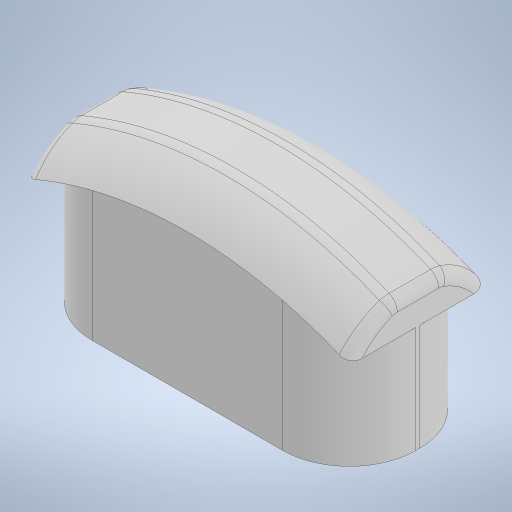
# Autodesk Inventor part: гриб
Saved by Autodesk Inventor 2023.1 (Build 271208000, 208)
## iProperties
Created: 2024-12-27
Part Number: гриб
Material: Типовые
Document SubType Name: Modeling
Designer: DELL
Density: 1 g/cm^3
Appearance: По умолчанию
Author: DELL
Autodesk Inventor part; units mm, degrees
ref_plane "YZ Plane" through (0, 0, 0) normal (1, 0, 0) x (0, 1, 0)
ref_plane "XZ Plane" through (0, 0, 0) normal (0, 1, 0) x (-1, 0, 0)
ref_plane "XY Plane" through (0, 0, 0) normal (0, 0, 1) x (1, 0, 0)
sketch "Эскиз1" plane through (0, 0, 0) normal (0, 1, 0) x (-1, 0, 0)
  line L0 (7.15, 2.15) -> (-7.15, 2.15)
  line L1 (-9.15, 0.15) -> (-9.15, -0.15)
  line L2 (-7.15, -2.15) -> (7.15, -2.15)
  line L3 (9.15, -0.15) -> (9.15, 0.15)
  line L4 (9.15, 2.15) -> (-9.15, -2.15) construction
  line L5 (-9.15, 2.15) -> (9.15, -2.15) construction
  arc A0 (-7.15, 2.15) -> (-9.15, 0.15) centre (-7.15, 0.15) ccw
  arc A1 (-9.15, -0.15) -> (-7.15, -2.15) centre (-7.15, -0.15) ccw
  arc A2 (9.15, 0.15) -> (7.15, 2.15) centre (7.15, 0.15) ccw
  arc A3 (7.15, -2.15) -> (9.15, -0.15) centre (7.15, -0.15) ccw
  line L6 (7.15, -5.15) -> (-7.15, -5.15)
  arc A4 (-12.15, -0.15) -> (-7.15, -5.15) centre (-7.15, -0.15) ccw
  line L7 (-12.15, -0.15) -> (-12.15, 0.15)
  arc A5 (-7.15, 5.15) -> (-12.15, 0.15) centre (-7.15, 0.15) ccw
  line L8 (-7.15, 5.15) -> (7.15, 5.15)
  arc A6 (12.15, 0.15) -> (7.15, 5.15) centre (7.15, 0.15) ccw
  line L9 (12.15, 0.15) -> (12.15, -0.15)
  arc A7 (7.15, -5.15) -> (12.15, -0.15) centre (7.15, -0.15) ccw
  point P0 (0, 0)
  dimension "d0" = 18.3
  dimension "d1" = 4.3
  dimension "d2" = 2
  dimension "d3" = 3
  constraints: 20 end point, 16 point on circle, 8 centre point, 8 point on line, 8 tangent, 4 parallel, 3 equal radius, 2 midpoint, 2 perpendicular, 1 horizontal, 7 other
  measures "d0" distance of L4.end L5.end
  measures "d1" distance of L5.start L4.end
  measures "d2" radius of A0
  measures "d3" distance between parallel lines of L2 L6
extrude "Выдавливание1" add sketch "Эскиз1" along normal blind 8
sketch "Эскиз2" plane through (12.15, 0, 0.15) normal (1, 0, 0) x (0, 0, -1)
  line L0 (0, 0) -> (0, 8) construction
  line L1 (0, 8) -> (0.3, 8) construction
  line L2 (0.3, 0) -> (0.3, 8) construction
  line L3 (0.3, 0) -> (0, 0) construction
  line L4 (-5, 0) -> (-5, 8) construction
  line L5 (5.3, 8) -> (0.3, 8) projected
  line L6 (-5, 8) -> (5.3, 8)
  line L7 (-1.4023, 10.3381) -> (1.7023, 10.3381)
  arc A0 (5.3, 8) -> (2.4133, 10.2075) centre (0.15, 4.2565) ccw
  arc A1 (-2.1133, 10.2075) -> (-5, 8) centre (0.15, 4.2565) ccw
  arc A2 (-1.4023, 10.3381) -> (-2.1133, 10.2075) centre (-1.4023, 8.3381) ccw
  arc A3 (2.4133, 10.2075) -> (1.7023, 10.3381) centre (1.7023, 8.3381) ccw
  point P0 (-1.7343, 10.3381)
  point P1 (2.0343, 10.3381)
  dimension "d6" = 2
  constraints: 14 end point, 10 point on circle, 4 centre point, 4 tangent, 2 horizontal, 2 point on line, 1 equal radius
  measures "d6" radius of A2
ref_plane "РабПлоскость1" through (-7.15, 0, 0) normal (0, 0, 1) x (1, 0, 0)
sketch "Эскиз3" plane through (-7.15, 0, 0) normal (0, 0, 1) x (1, 0, 0)
  line L0 (19.3, 8) -> (19.3, 10.2075) construction
  line L1 (0, 0) -> (-5, 0) projected
  line L2 (-5, 0) -> (-5, 15.3004) construction
  arc A0 (19.3, 9.1037) -> (-5, 9.1037) centre (7.15, -17.7297) ccw
  point P0 (7.15, 0)
  constraints: 2 end point, 2 point on circle, 1 centre point, 1 midpoint, 1 point on line, 1 vertical
sweep "Сдвиг1" add profiles "Эскиз2" path "Эскиз3" keep normal constant yes path curves A0
sketch "Эскиз4" plane through (0, 8, 0) normal (0, 1, 0) x (1, 0, 0)
  line L0 (-7.15, -5.15) -> (7.15, -5.15)
  arc A0 (-12.15, -0.15) -> (-7.15, -5.15) centre (-7.15, -0.15) ccw
  line L1 (-12.15, 0.15) -> (-12.15, -0.15)
  arc A1 (-7.15, 5.15) -> (-12.15, 0.15) centre (-7.15, 0.15) ccw
  line L2 (7.15, 5.15) -> (-7.15, 5.15)
  arc A2 (12.15, 0.15) -> (7.15, 5.15) centre (7.15, 0.15) ccw
  line L3 (12.15, -0.15) -> (12.15, 0.15)
  arc A3 (7.15, -5.15) -> (12.15, -0.15) centre (7.15, -0.15) ccw
  arc A4 (-9.15, -0.15) -> (-7.15, -2.15) centre (-7.15, -0.15) ccw
  line L4 (7.15, -2.15) -> (-7.15, -2.15)
  arc A5 (7.15, -2.15) -> (9.15, -0.15) centre (7.15, -0.15) ccw
  line L5 (9.15, 0.15) -> (9.15, -0.15)
  arc A6 (9.15, 0.15) -> (7.15, 2.15) centre (7.15, 0.15) ccw
  line L6 (-7.15, 2.15) -> (7.15, 2.15)
  arc A7 (-7.15, 2.15) -> (-9.15, 0.15) centre (-7.15, 0.15) ccw
  line L7 (-9.15, -0.15) -> (-9.15, 0.15)
  line L8 (10.65, 0.15) -> (10.65, -0.15)
  line L9 (-10.65, -0.15) -> (-10.65, 0.15)
  point P0 (0, 0)
  dimension "d1" = 4.3
  constraints: 20 end point, 16 centre point, 16 point on circle
extrude "Выдавливание3" add sketch "Эскиз4" along normal up to surface round surface about axis through (0, -18.8334, 5.15) along (0, 0, 1) radius 29.456 far side no
fillet "Сопряжение1" radius 1 10 edges at (-12.15, 10.3052, 1.9138) (-12.15, 10.3381, 0) (-12.15, 10.3052, -1.9138) (-12.15, 9.3141, -3.8675) (-12.15, 9.3141, 3.8675) (12.15, 10.3052, 1.9138) (12.15, 10.3381, 0) (12.15, 10.3052, -1.9138) (12.15, 9.3141, -3.8675) (12.15, 9.3141, 3.8675)
